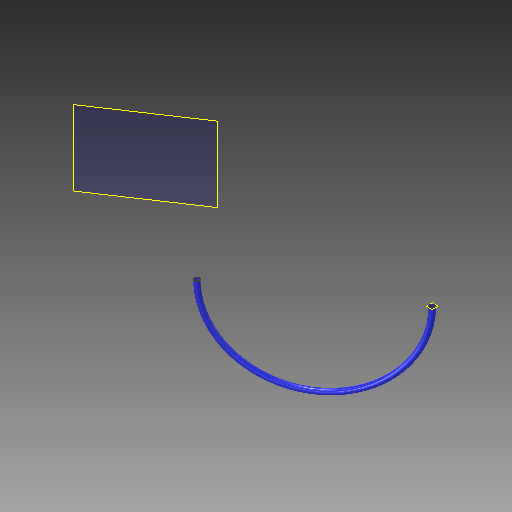
# Autodesk Inventor part: winding_not_formed_1_A
Saved by Autodesk Inventor 2018 (Build 220112000, 112)
## iProperties
Created: 2017-07-07
Part Number: winding_not_formed_1_A
Material: Типовые
Document SubType Name: Modeling
Designer: user
Density: 1 g/cm^3
Appearance: По умолчанию
Author: user
Autodesk Inventor part; units mm, degrees
ref_plane "YZ Plane" through (0, 0, 0) normal (1, 0, 0) x (0, 1, 0)
ref_plane "XZ Plane" through (0, 0, 0) normal (0, 1, 0) x (-1, 0, 0)
ref_plane "XY Plane" through (0, 0, 0) normal (0, 0, 1) x (1, 0, 0)
ref_plane "РабПлоскость1" through (151.1609, -132.5604, -259.1713) normal (-0.5555702, 0, -0.8314696) x (0, -1, 0)
sketch "Эскиз2" plane through (151.1609, -132.5604, -259.1713) normal (-0.5555702, 0, -0.8314696) x (0, -1, 0)
  arc A0 (0, 0) -> (0, 221.6282) centre (0, 110.8141) ccw
  point P0 (-132.5604, 269.6735)
  constraints: 2 point on circle, 1 centre point
ref_plane "РабПлоскость2" through (151.1609, -132.5604, -259.1713) normal (0, -1, 0) x (1, 0, 0)
sketch "Эскиз3" plane through (151.1609, -132.5604, -259.1713) normal (0, -1, 0) x (1, 0, 0)
  circle A0 centre (0, 0) radius 3.5 projected
  circle A1 centre (0, 0) radius 2.5 projected
  circle A2 centre (0, 0) radius 1.75 projected
  point P0 (-151.1609, 259.1713)
sweep "Сдвиг1" add profiles "Эскиз3" path "Эскиз2" contours A0
